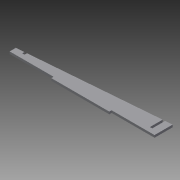
# Autodesk Inventor part: angle_plate_long_short
Saved by Autodesk Inventor 2015 SP1 (Build 190203100, 203)
## iProperties
Created: 2016-08-03
Part Number: angle_plate_long_short
Material: Generic
Document SubType Name: Modeling
Designer: polidorop
Density: 1 g/cm^3
Appearance: Default
Author: polidorop
Autodesk Inventor part; units mm, degrees
ref_plane "YZ Plane" through (0, 0, 0) normal (1, 0, 0) x (0, 1, 0)
ref_plane "XZ Plane" through (0, 0, 0) normal (0, 1, 0) x (-1, 0, 0)
ref_plane "XY Plane" through (0, 0, 0) normal (0, 0, 1) x (1, 0, 0)
sketch "Sketch1" plane through (0, 0, 0) normal (0, 0, 1) x (1, 0, 0)
  line L0 (-64, 50) -> (64, 50)
  line L1 (64, 50) -> (64, 0)
  line L2 (64, 0) -> (-64, 0)
  line L3 (-64, 0) -> (-64, 50)
  line L4 (-25, 0) -> (25, 0)
  line L5 (25, 0) -> (25, -2)
  line L6 (25, -2) -> (-25, -2)
  line L7 (-25, -2) -> (-25, 0)
  point P0 (0, 0)
  point P1 (0, 0)
  dimension "d0" = 50
  dimension "d1" = 128
  dimension "d2" = 2
  dimension "d3" = 50
  constraints: 16 end point, 4 parallel, 2 horizontal, 2 midpoint, 2 perpendicular, 1 coincident
  measures "d0" distance of L2.end L0.start
  measures "d1" distance of L0.start L0.end
  measures "d2" distance of L6.end L4.start
  measures "d3" distance of L5.end L6.end
extrude "Extrusion1" add sketch "Sketch1" along normal mid plane 2
sketch "Sketch2" plane through (0, 0, 1) normal (0, 0, 1) x (1, 0, 0)
  line L0 (53.9533, 19.1647) -> (54.2948, 15.001) projected
  line L1 (54.2948, 15.001) -> (-55.3369, 6.0072) projected
  line L2 (-55.3369, 6.0072) -> (-55.6784, 10.1709) projected
  line L3 (-55.6784, 10.1709) -> (53.9533, 19.1647) projected
  line L4 (62.1376, 13.5765) -> (61.7855, 17.8679) projected
  line L5 (-63.1946, 7.615) -> (-62.8426, 3.3235) projected
  point P0 (0, 0)
sketch "Sketch3" plane through (0, 0, 1) normal (0, 0, 1) x (1, 0, 0)
  line L0 (-63.1946, 7.615) -> (-62.8426, 3.3235) construction
  line L1 (62.1376, 13.5765) -> (61.7855, 17.8679) construction
  line L2 (54.2948, 15.001) -> (-55.3369, 6.0072) construction
  line L3 (-62.8426, 5.3914) -> (61.9691, 15.6306)
  line L4 (-62.8426, 5.3914) -> (-62.8426, 0)
  line L5 (-62.8426, 0) -> (-72.8426, 0)
  line L6 (-72.8426, 0) -> (-72.8426, 60)
  line L7 (-72.8426, 60) -> (71.9691, 60)
  line L8 (71.9691, 60) -> (71.9691, 0)
  line L9 (71.9691, 0) -> (61.9691, 0)
  line L10 (61.9691, 0) -> (61.9691, 15.6306)
  point P0 (0, 0)
  dimension "d6" = 10
  dimension "d7" = 60
  dimension "d8" = 10
  constraints: 16 end point, 5 perpendicular, 5 point on line, 1 collinear, 1 vertical
  measures "d6" distance of L4.end L5.end
  measures "d7" distance of L5.end L6.end
  measures "d8" distance of L8.end L9.end
extrude "Extrusion2" cut sketch "Sketch3" against normal through all
sketch "Sketch4" plane through (0, 0, 1) normal (0, 0, 1) x (1, 0, 0)
  line L0 (56, 14.7768) -> (56, 0) projected
  line L1 (54, 14.7768) -> (56, 14.7768) projected
  line L2 (54, 0) -> (54, 14.7768) projected
  line L3 (56, 0) -> (54, 0) projected
  line L4 (-54, 5.783) -> (-54, 0) projected
  line L5 (-56, 5.783) -> (-54, 5.783) projected
  line L6 (-56, 0) -> (-56, 5.783) projected
  line L7 (-54, 0) -> (-56, 0) projected
  point P0 (0, 0)
sketch "Sketch5" plane through (0, 0, 1) normal (0, 0, 1) x (1, 0, 0)
  line L0 (-56, 0) -> (-56, 5.783) construction
  line L1 (-54, 5.783) -> (-54, 0) construction
  line L2 (54, 0) -> (54, 14.7768) construction
  line L3 (56, 14.7768) -> (56, 0) construction
  line L4 (-54, 4) -> (-56, 4)
  line L5 (-56, 4) -> (-56, 24)
  line L6 (-56, 24) -> (-54, 24)
  line L7 (-54, 24) -> (-54, 4)
  line L8 (56, 24) -> (54, 24)
  line L9 (54, 24) -> (54, 4)
  line L10 (54, 4) -> (56, 4)
  line L11 (56, 4) -> (56, 24)
  line L12 (-62.8426, 0) -> (-25, 0) projected
  line L13 (25, 0) -> (61.9691, 0) projected
  point P0 (0, 0)
  dimension "d11" = 4
  dimension "d12" = 20
  dimension "d13" = 4
  dimension "d14" = 20
  constraints: 16 end point, 4 parallel, 4 point on line, 2 horizontal, 2 perpendicular
  measures "d11" distance between parallel lines of L12 L4
  measures "d12" distance between parallel lines of L4 L6
  measures "d13" distance between parallel lines of L13 L10
  measures "d14" distance between parallel lines of L10 L8
extrude "Extrusion3" cut sketch "Sketch5" against normal through all
body "Solid1"
